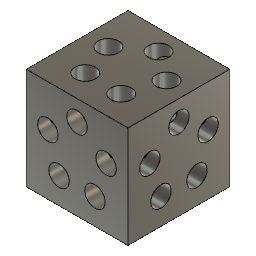
Semana3_Desafio5 v1 (Autodesk Fusion 360 design; units mm, degrees)
Autodesk Fusion 360 part; units mm, degrees
sketch "Sketch1" plane through (0, 0, 0) normal (0, 0, 1) x (1, 0, 0)
  line L0 (25, 25) -> (-25, 25)
  line L1 (-25, 25) -> (-25, -25)
  line L2 (-25, -25) -> (25, -25)
  line L3 (25, -25) -> (25, 25)
  line L4 (25, 25) -> (-25, -25) construction
  line L5 (-25, 25) -> (25, -25) construction
  dimension "d1" = 50
  dimension "d2" = 50
  constraint horizontal L0
  constraint perpendicular L0 L1
  constraint parallel L0 L2
  constraint parallel L1 L3
  constraint coincident L4 origin
  constraint coincident L5 origin
  measures "d1" distance of L1.end L2.end
  measures "d2" distance of L0.end L1.end
extrude "Extrude1" add sketch "Sketch1" along normal mid plane 50
sketch "Sketch2" plane through (0, 0, 25) normal (0, 0, 1) x (-1, 0, 0)
  line L0 (-25, 25) -> (-25, -25)
  line L1 (-25, -25) -> (25, -25)
  line L2 (25, -25) -> (25, 25)
  line L3 (25, 25) -> (-25, 25)
  circle A0 centre (0, -15) radius 5
  dimension "d5" = 10
  measures "d5" diameter of A0
extrude "Extrude2" cut sketch "Sketch2" against normal through all contours A0
pattern_circular "C-Pattern1" count 5 over 360 about axis through (0, 0, 1.75) along (0, 0, 1) of "Extrude2"
sketch "Sketch3" plane through (25, 0, 0) normal (1, 0, 0) x (0, 1, 0)
  line L0 (25, -25) -> (25, 25)
  line L1 (25, 25) -> (-25, 25)
  line L2 (-25, 25) -> (-25, -25)
  line L3 (-25, -25) -> (25, -25)
  circle A0 centre (0, 15) radius 5
  dimension "d9" = 10
  measures "d9" diameter of A0
extrude "Extrude3" cut sketch "Sketch3" against normal through all contours A0
pattern_circular "C-Pattern2" count 5 over 360 about axis through (1.75, 0, 0) along (1, 0, 0) of "Extrude3"
sketch "Sketch4" plane through (0, -25, 0) normal (0, -1, 0) x (1, 0, 0)
  line L0 (25, -25) -> (25, 25)
  line L1 (25, 25) -> (-25, 25)
  line L2 (-25, 25) -> (-25, -25)
  line L3 (-25, -25) -> (25, -25)
  circle A0 centre (0, 15) radius 5
  dimension "d13" = 10
  measures "d13" diameter of A0
extrude "Extrude4" cut sketch "Sketch4" against normal through all contours A0
pattern_circular "C-Pattern3" count 5 over 360 about axis through (0, 1.75, 0) along (0, 1, 0) of "Extrude4"
